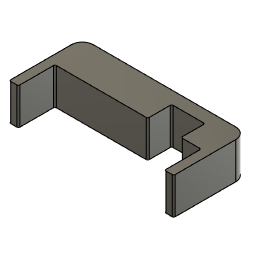
MGN9_rail_guide_DOOM_4040 v1 (Autodesk Fusion 360 design; units mm, degrees)
Autodesk Fusion 360 part; units mm, degrees
sketch "Sketch1" plane through (0, 0, 0) normal (0, 1, 0) x (1, 0, 0)
  line L0 (-22.5, 10) -> (22.5, 10)
  line L1 (22.5, 10) -> (22.5, -10)
  line L2 (22.5, -10) -> (-22.5, -10)
  line L3 (-22.5, -10) -> (-22.5, 10)
  line L4 (-22.5, 10) -> (22.5, -10) construction
  line L5 (22.5, 10) -> (-22.5, -10) construction
  dimension "d1" = 45
  dimension "d2" = 20
  constraint horizontal L0
  constraint perpendicular L0 L1
  constraint parallel L0 L2
  constraint parallel L1 L3
  constraint coincident L4 origin
  constraint coincident L5 origin
  measures "d1" distance of L1.end L2.end
  measures "d2" distance of L0.end L1.end
extrude "Extrude1" add sketch "Sketch1" along normal blind 10
sketch "Sketch2" plane through (0, 10, 0) normal (0, 1, 0) x (-1, 0, 0)
  line L0 (22.5, 10) -> (-22.5, 10)
  line L1 (-22.5, 10) -> (-22.5, -10)
  line L2 (-22.5, -10) -> (22.5, -10)
  line L3 (22.5, -10) -> (22.5, 10)
  line L4 (20, 10) -> (-20, 10)
  line L5 (-20, 10) -> (-20, 0)
  line L6 (-20, 0) -> (20, 0)
  line L7 (20, 0) -> (20, 10)
  dimension "d5" = 40
  dimension "d6" = 10
  dimension "d7" = 2.5
  constraint horizontal L4
  constraint vertical L5
  constraint horizontal L6
  constraint vertical L7
  constraint coincident L0 L4.start
  measures "d5" distance of L4.start L4.end
  measures "d6" distance of L4.start L6.end
  measures "d7" distance of L0.start L4.start
extrude "Extrude2" cut sketch "Sketch2" against normal through all contours L0 L4 L5 L6 L7
sketch "Sketch3" plane through (0, 10, 0) normal (0, 1, 0) x (-1, 0, 0)
  line L0 (20, 10) -> (20, 0)
  line L1 (20, 0) -> (-20, 0)
  line L2 (-20, 0) -> (-20, 10)
  line L3 (-20, 10) -> (-22.5, 10)
  line L4 (-22.5, 10) -> (-22.5, -10)
  line L5 (-22.5, -10) -> (22.5, -10)
  line L6 (22.5, -10) -> (22.5, 10)
  line L7 (22.5, 10) -> (20, 10)
  line L8 (-14.5, 0) -> (-5.4, 0)
  line L9 (-5.4, 0) -> (-5.4, -6.55)
  line L10 (-5.4, -6.55) -> (-14.5, -6.55)
  line L11 (-14.5, -6.55) -> (-14.5, 0)
  dimension "d9" = 9.1
  dimension "d12" = 6.55
  dimension "d13" = 5.5
  constraint horizontal L8
  constraint vertical L9
  constraint horizontal L10
  constraint vertical L11
  constraint coincident L1 L8.start
  measures "d9" distance of L8.start L8.end
  measures "d12" distance of L8 L10
  measures "d13" distance of L1.end L8.start
extrude "Extrude3" cut sketch "Sketch3" against normal through all contours L1 L8 L9 L10 L11
fillet "Fillet1" radius 0.4 10 edges at (-20, 5, 10) (-20, 5, 0) (5.4, 5, 0) (5.4, 5, -6.55) (14.5, 5, -6.55) (14.5, 5, 0) (20, 5, 0) (20, 5, 10) (-22.5, 5, 10) (22.5, 5, 10)
fillet "Fillet2" radius 3 2 edges at (-22.5, 5, -10) (22.5, 5, -10)
